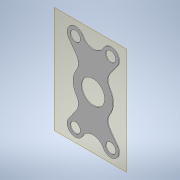
# Autodesk Inventor part: screw case gasket
Saved by Autodesk Inventor 2022 (Build 260153000, 153)
## iProperties
Created: 2022-11-12
Part Number: screw case gasket
Material: Generic
Document SubType Name: Modeling
Designer: efred
Density: 1 g/cm^3
Appearance: Default
Author: efred
Autodesk Inventor part; units mm, degrees
ref_plane "YZ Plane" through (0, 0, 0) normal (1, 0, 0) x (0, 1, 0)
ref_plane "XZ Plane" through (0, 0, 0) normal (0, 1, 0) x (-1, 0, 0)
ref_plane "XY Plane" through (0, 0, 0) normal (0, 0, 1) x (1, 0, 0)
ref_plane "Work Plane1" through (0, 0, 0) normal (0, 0, 1) x (1, 0, 0)
sketch "Sketch1" plane through (0, 0, 0) normal (0, 0, 1) x (1, 0, 0)
  circle A0 centre (0, 0) radius 5.3 construction
  circle A1 centre (-8, 17.9) radius 2.3 projected
  circle A2 centre (-8, -17.9) radius 2.3 projected
  circle A3 centre (8, -17.9) radius 2.3 projected
  circle A4 centre (8, 17.9) radius 2.3 projected
  arc A5 (4.4444, -19.7325) -> (11.2421, -15.5572) centre (8, -17.9) ccw projected
  line L0 (11.2421, -15.5572) -> (7.847, -10.8589) projected
  arc A6 (7.7389, -5.1575) -> (7.847, -10.8589) centre (11.8996, -7.9303) ccw projected
  arc A7 (-7.7389, 5.1575) -> (-7.7389, -5.1575) centre (0, 0) ccw projected
  arc A8 (7.847, 10.8589) -> (7.7389, 5.1575) centre (11.8996, 7.9303) ccw projected
  line L1 (7.847, 10.8589) -> (11.2421, 15.5572) projected
  arc A9 (11.2421, 15.5572) -> (4.4444, 19.7325) centre (8, 17.9) ccw projected
  arc A10 (-4.4444, 19.7325) -> (4.4444, 19.7325) centre (0, 22.0231) ccw projected
  arc A11 (-4.4444, 19.7325) -> (-11.2421, 15.5572) centre (-8, 17.9) ccw projected
  line L2 (-11.2421, 15.5572) -> (-7.847, 10.8589) projected
  arc A12 (-7.7389, 5.1575) -> (-7.847, 10.8589) centre (-11.8996, 7.9303) ccw projected
  arc A13 (-7.847, -10.8589) -> (-7.7389, -5.1575) centre (-11.8996, -7.9303) ccw projected
  line L3 (-7.847, -10.8589) -> (-11.2421, -15.5572) projected
  arc A14 (-11.2421, -15.5572) -> (-4.4444, -19.7325) centre (-8, -17.9) ccw projected
  arc A15 (4.4444, -19.7325) -> (-4.4444, -19.7325) centre (0, -22.0231) ccw projected
  line L4 (10.9989, 15.7329) -> (7.6038, 11.0346)
  arc A16 (7.6038, 11.0346) -> (7.4892, 4.9911) centre (11.8996, 7.9303) ccw
  arc A17 (7.4892, -4.9911) -> (7.4892, 4.9911) centre (0, 0) ccw
  arc A18 (7.4892, -4.9911) -> (7.6038, -11.0346) centre (11.8996, -7.9303) ccw
  line L5 (7.6038, -11.0346) -> (10.9989, -15.7329)
  arc A19 (4.7111, -19.5951) -> (10.9989, -15.7329) centre (8, -17.9) ccw
  arc A20 (4.7111, -19.5951) -> (-4.7111, -19.5951) centre (0, -22.0231) ccw
  arc A21 (-10.9989, -15.7329) -> (-4.7111, -19.5951) centre (-8, -17.9) ccw
  line L6 (-10.9989, -15.7329) -> (-7.6038, -11.0346)
  arc A22 (-7.6038, -11.0346) -> (-7.4892, -4.9911) centre (-11.8996, -7.9303) ccw
  arc A23 (-7.4892, 4.9911) -> (-7.4892, -4.9911) centre (0, 0) ccw
  arc A24 (-7.4892, 4.9911) -> (-7.6038, 11.0346) centre (-11.8996, 7.9303) ccw
  line L7 (-7.6038, 11.0346) -> (-10.9989, 15.7329)
  arc A25 (-4.7111, 19.5951) -> (-10.9989, 15.7329) centre (-8, 17.9) ccw
  arc A26 (-4.7111, 19.5951) -> (4.7111, 19.5951) centre (0, 22.0231) ccw
  arc A27 (10.9989, 15.7329) -> (4.7111, 19.5951) centre (8, 17.9) ccw
  circle A28 centre (0, 0) radius 3.8 projected
  circle A29 centre (0, 0) radius 4
  arc A30 (7.7389, -5.1575) -> (7.7389, 5.1575) centre (0, 0) ccw projected
  point P0 (0, 0)
  point P1 (11.8996, -7.9303)
  point P2 (11.8996, 7.9303)
  point P3 (11.8996, -7.9303)
  point P4 (11.8996, 7.9303)
  dimension "d0" = 0.3
  dimension "d3" = 0.2
  constraints: 24 point on circle, 13 centre point, 8 end point, 13 other
  measures "d0" distance between parallel lines of L1 L4
  measures "d3" radial gap between concentric circles of A28 A29
extrude "Extrusion1" add sketch "Sketch1" along normal blind 0.3 contours L4 A16 A17 A18 L5 A19 A20 A21 L6 A22 A23 A24 L7 A25 A26 A27
body "Solid1"
